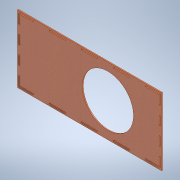
# Autodesk Inventor part: Pieza agujero
Saved by Autodesk Inventor 2020.2 (Build 242310000, 310)
## iProperties
Created: 2020-04-18
Part Number: Pieza agujero
Material: Madera (nogal)
Document SubType Name: Modeling
Designer: miosh
Density: 0.55 g/cm^3
Appearance: Nogal - Natural pulido
Author: miosh
Autodesk Inventor part; units mm, degrees
ref_plane "YZ Plane" through (0, 0, 0) normal (1, 0, 0) x (0, 1, 0)
ref_plane "XZ Plane" through (0, 0, 0) normal (0, 1, 0) x (-1, 0, 0)
ref_plane "XY Plane" through (0, 0, 0) normal (0, 0, 1) x (1, 0, 0)
sketch "Boceto1" plane through (0, 0, 0) normal (0, 0, 1) x (1, 0, 0)
  line L0 (0, 0) -> (0, 210)
  line L1 (0, 210) -> (450, 210)
  line L2 (450, 210) -> (450, 0)
  line L3 (450, 0) -> (0, 0)
  line L4 (0, 210) -> (5, 210)
  line L5 (5, 205) -> (50, 205)
  line L6 (50, 205) -> (50, 202)
  line L7 (5, 205) -> (5, 174.29)
  line L8 (5, 174.29) -> (8, 174.29)
  line L9 (8, 174.29) -> (8, 202)
  line L10 (8, 202) -> (50, 202)
  line L11 (0, 0) -> (5, 0)
  line L12 (0, 0) -> (5, 0)
  line L13 (5, 5) -> (50, 5)
  line L14 (5, 5) -> (5, 35.71)
  line L15 (5, 35.71) -> (8, 35.71)
  line L16 (50, 5) -> (50, 8)
  line L17 (8, 35.71) -> (8, 8)
  line L18 (8, 8) -> (50, 8)
  line L19 (450, 0) -> (445, 0)
  line L20 (445, 5) -> (445, 35.71)
  line L21 (445, 35.71) -> (442, 35.71)
  line L22 (445, 5) -> (400, 5)
  line L23 (400, 5) -> (400, 8)
  line L24 (400, 8) -> (442, 8)
  line L25 (442, 8) -> (442, 35.71)
  line L26 (450, 210) -> (445, 210)
  line L27 (445, 205) -> (400, 205)
  line L28 (445, 205) -> (445, 174.29)
  line L29 (445, 174.29) -> (442, 174.29)
  line L30 (400, 205) -> (400, 202)
  line L31 (400, 202) -> (442, 202)
  line L32 (442, 202) -> (442, 174.29)
  line L33 (5, 63.43) -> (5, 91.14)
  line L34 (5, 91.14) -> (8, 91.14)
  line L35 (8, 91.14) -> (8, 63.43)
  line L36 (8, 63.43) -> (5, 63.43)
  line L37 (5, 118.86) -> (5, 146.57)
  line L38 (5, 118.86) -> (8, 118.86)
  line L39 (8, 118.86) -> (8, 146.57)
  line L40 (8, 146.57) -> (5, 146.57)
  line L41 (445, 63.43) -> (445, 91.14)
  line L42 (445, 63.43) -> (442, 63.43)
  line L43 (442, 63.43) -> (442, 91.14)
  line L44 (442, 91.14) -> (445, 91.14)
  line L45 (445, 118.86) -> (442, 118.86)
  line L46 (442, 118.86) -> (442, 146.57)
  line L47 (442, 146.57) -> (445, 146.57)
  line L48 (445, 146.57) -> (445, 118.86)
  line L49 (350, 205) -> (300, 205)
  line L50 (300, 205) -> (300, 202)
  line L51 (300, 202) -> (350, 202)
  line L52 (350, 202) -> (350, 205)
  line L53 (250, 205) -> (200, 205)
  line L54 (200, 205) -> (200, 202)
  line L55 (200, 202) -> (250, 202)
  line L56 (250, 202) -> (250, 205)
  line L57 (150, 205) -> (100, 205)
  line L58 (100, 205) -> (100, 202)
  line L59 (100, 202) -> (150, 202)
  line L60 (150, 202) -> (150, 205)
  line L61 (350, 8) -> (300, 8)
  line L62 (300, 8) -> (300, 5)
  line L63 (300, 5) -> (350, 5)
  line L64 (350, 5) -> (350, 8)
  line L65 (250, 8) -> (200, 8)
  line L66 (200, 8) -> (200, 5)
  line L67 (200, 5) -> (250, 5)
  line L68 (250, 5) -> (250, 8)
  line L69 (150, 8) -> (100, 8)
  line L70 (100, 8) -> (100, 5)
  line L71 (100, 5) -> (150, 5)
  line L72 (150, 5) -> (150, 8)
  point P0 (450, 30)
  dimension "d8" = 210
  dimension "d9" = 210
  dimension "d10" = 5
  dimension "d11" = 27.72
  dimension "d12" = 5
  dimension "d13" = 5
  dimension "d14" = 450
  dimension "d15" = 5
  dimension "d16" = 5
  dimension "d17" = 5
  dimension "d18" = 45
  dimension "d19" = 30.71
  dimension "d20" = 3
  dimension "d21" = 3
  dimension "d22" = 30.71
  dimension "d23" = 45
  dimension "d24" = 3
  dimension "d25" = 3
  dimension "d26" = 5
  dimension "d27" = 5
  dimension "d29" = 5
  dimension "d30" = 30.71
  dimension "d31" = 45
  dimension "d32" = 5
  dimension "d33" = 3
  dimension "d34" = 3
  dimension "d35" = 5
  dimension "d36" = 5
  dimension "d37" = 45
  dimension "d38" = 30.71
  dimension "d39" = 3
  dimension "d40" = 3
  dimension "d41" = 50
  dimension "d42" = 5
  dimension "d43" = 5
  dimension "d44" = 5
  dimension "d45" = 3
  dimension "d46" = 3
  constraints: 146 end point, 32 perpendicular, 15 horizontal, 10 vertical, 5 point on line, 2 parallel, 1 collinear
  measures "d8" distance of L26.start L19.start
  measures "d9" distance of L11.start L4.start
  measures "d10" distance between parallel lines of L0 L33
  measures "d11" distance of L33.start L15.start
  measures "d12" distance between parallel lines of L0 L37
  measures "d13" distance between parallel lines of L0 L7
  measures "d14" distance of L4.start L26.start
  measures "d15" distance between parallel lines of L1 L5
  measures "d16" distance between parallel lines of L1 L57
  measures "d17" distance between parallel lines of L1 L53
  measures "d18" distance of L5.start L6.start
  measures "d19" distance of L5.start L8.start
  measures "d20" distance of L6.start L6.end
  measures "d21" distance of L8.start L8.end
  measures "d22" distance of L14.start L15.start
  measures "d23" distance of L14.start L16.start
  measures "d24" distance of L16.start L16.end
  measures "d25" distance of L15.start L15.end
  measures "d26" distance between parallel lines of L3 L13
  measures "d27" distance between parallel lines of L0 L14
  measures "d29" distance between parallel lines of L2 L20
  measures "d30" distance of L20.start L20.end
  measures "d31" distance of L20.start L22.end
  measures "d32" distance between parallel lines of L3 L22
  measures "d33" distance of L22.end L23.end
  measures "d34" distance of L20.end L21.end
  measures "d35" distance between parallel lines of L2 L28
  measures "d36" distance between parallel lines of L27 L1
  measures "d37" distance of L28.start L27.end
  measures "d38" distance of L28.start L29.start
  measures "d39" distance of L27.end L31.start
  measures "d40" distance of L29.start L29.end
  measures "d41" distance of L70.start L16.end
  measures "d42" distance between parallel lines of L3 L71
  measures "d43" distance between parallel lines of L3 L67
  measures "d44" distance between parallel lines of L3 L63
  measures "d45" distance of L61.end L62.end
  measures "d46" distance of L71.end L69.start
sketch "Boceto2" plane through (0, 0, 0) normal (0, 0, 1) x (1, 0, 0)
  line L0 (449.8604, 0) -> (282.2704, 0)
  circle A0 centre (282.2704, 105) radius 80
  point P0 (0, 0)
  constraints: 2 end point, 1 centre point, 1 horizontal
extrude "Extrusión1" add sketch "Boceto1" along normal blind 3
extrude "Extrusión2" cut sketch "Boceto2" along normal blind 3
